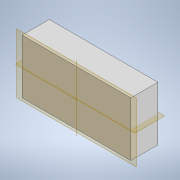
# Autodesk Inventor part: FootP_flat
Saved by Autodesk Inventor 2021 (Build 250183000, 183)
## iProperties
Created: 2020-12-19
Part Number: FootP_flat
Material: 一般
Document SubType Name: Modeling
Designer: Tazaki
Density: 0.865039 g/cm^3
Appearance: 既定
Mass: 500 g
Surface Area: 470 cm^2
Volume: 600 cm^3
Author: Tazaki
Autodesk Inventor part; units mm, degrees
ref_plane "YZ Plane" through (0, 0, 0) normal (1, 0, 0) x (0, 1, 0)
sketch "スケッチ2" plane through (0, 0, 0) normal (0, 0, 1) x (1, 0, 0)
  line L0 (-100, 50) -> (100, 50)
  line L1 (100, 50) -> (100, -50)
  line L2 (100, -50) -> (-100, -50)
  line L3 (-100, -50) -> (-100, 50)
  point P0 (0, 0)
  point P1 (-100, 0)
  dimension "d2" = 200
  dimension "d3" = 100
  dimension "d4" = 100
  constraints: 8 end point, 2 parallel, 1 horizontal, 1 horizontal alignment, 1 midpoint, 1 perpendicular
  measures "d2" distance of L0.start L0.end
  measures "d3" distance of L2.end L0.start
  measures "d4" distance from line of point (0, 0) L3
extrude "押し出し1" add sketch "スケッチ2" against normal blind 50
